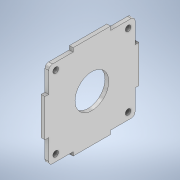
# Autodesk Inventor part: UpperSide
Saved by Autodesk Inventor 2022 (Build 260153000, 153)
## iProperties
Created: 2022-04-02
Part Number: UpperSide
Material: Aluminum 6061, Welded
Document SubType Name: Modeling
Designer: Sergei
Density: 2.7 g/cm^3
Appearance: Aluminum - Polished
Author: Sergei
Autodesk Inventor part; units mm, degrees
ref_plane "YZ Plane" through (0, 0, 0) normal (1, 0, 0) x (0, 1, 0)
ref_plane "XZ Plane" through (0, 0, 0) normal (0, 1, 0) x (-1, 0, 0)
ref_plane "XY Plane" through (0, 0, 0) normal (0, 0, 1) x (1, 0, 0)
sketch "Sketch1" plane through (0, 0, 0) normal (1, 0, 0) x (0, 1, 0)
  line L0 (-25, -25) -> (25, -25)
  line L1 (25, -25) -> (25, 25)
  line L2 (25, 25) -> (-25, 25)
  line L3 (-25, 25) -> (-25, -25)
  line L4 (-25, -25) -> (25, 25) construction
  line L5 (25, -25) -> (-25, 25) construction
  line L6 (-24, -24) -> (24, -24)
  line L7 (24, -24) -> (24, 24)
  line L8 (24, 24) -> (-24, 24)
  line L9 (-24, 24) -> (-24, -24)
  line L10 (-24, -24) -> (24, 24) construction
  line L11 (24, -24) -> (-24, 24) construction
  point P0 (0, 0)
  dimension "d0" = 50
  dimension "d1" = 50
  dimension "d2" = 48
  dimension "d3" = 48
  constraints: 24 end point, 4 midpoint, 4 parallel, 2 horizontal, 2 perpendicular, 1 point on line
  measures "d0" distance of L0.end L1.end
  measures "d1" distance of L0.start L0.end
  measures "d2" distance of L6.end L7.end
  measures "d3" distance of L6.start L6.end
extrude "Extrusion1" add sketch "Sketch1" along normal blind 2 contours L3 L2 L1 L0 | L9 L8 L7 L6
sketch "Sketch3" plane through (0, 0, 0) normal (-1, 0, 0) x (0, 0, 1)
  line L0 (19.3, -19.3) -> (-19.3, -19.3)
  line L1 (-19.3, -19.3) -> (-19.3, 19.3)
  line L2 (-19.3, 19.3) -> (19.3, 19.3)
  line L3 (19.3, 19.3) -> (19.3, -19.3)
  line L4 (19.3, -19.3) -> (-19.3, 19.3) construction
  line L5 (-19.3, -19.3) -> (19.3, 19.3) construction
  circle A0 centre (-19.3, 19.3) radius 1.5
  circle A1 centre (19.3, 19.3) radius 1.5555
  circle A2 centre (19.3, -19.3) radius 1.5555
  circle A3 centre (-19.3, -19.3) radius 1.5555
  point P0 (0, 0)
  dimension "d6" = 38.6
  dimension "d7" = 38.6
  dimension "d8" = 3
  dimension "d9" = 3.111
  dimension "d10" = 3.111
  dimension "d11" = 3.111
  constraints: 12 end point, 4 centre point, 4 coincident, 2 midpoint, 2 parallel, 1 horizontal, 1 perpendicular
  measures "d6" distance of L1.end L2.end
  measures "d7" distance of L2.end L0.start
  measures "d8" diameter of A0
  measures "d9" diameter of A1
  measures "d10" diameter of A2
  measures "d11" diameter of A3
hole "Hole1" at (0, 19.3, -19.3) direction (1, 0, 0) diameter 3 end through all
sketch "Sketch4" plane through (0, 0, 0) normal (-1, 0, 0) x (0, 0, 1)
  line L0 (-19.3, -19.3) -> (19.3, -19.3)
  line L1 (19.3, -19.3) -> (19.3, 19.3)
  line L2 (19.3, 19.3) -> (-19.3, 19.3)
  line L3 (-19.3, 19.3) -> (-19.3, -19.3)
  line L4 (-19.3, -19.3) -> (19.3, 19.3) construction
  line L5 (19.3, -19.3) -> (-19.3, 19.3) construction
  circle A0 centre (19.3, 19.3) radius 1.5
  point P0 (0, 0)
  dimension "d19" = 38.6
  dimension "d20" = 38.6
  dimension "d21" = 3
  constraints: 12 end point, 2 midpoint, 2 parallel, 1 centre point, 1 horizontal, 1 perpendicular, 1 point on line
  measures "d19" distance of L0.end L1.end
  measures "d20" distance of L0.start L0.end
  measures "d21" diameter of A0
hole "Hole2" at (0, 19.3, 19.3) direction (1, 0, 0) diameter 3 end through all
sketch "Sketch5" plane through (0, 0, 0) normal (-1, 0, 0) x (0, 0, 1)
  line L0 (19.3, -19.3) -> (-19.3, -19.3)
  line L1 (-19.3, -19.3) -> (-19.3, 19.3)
  line L2 (-19.3, 19.3) -> (19.3, 19.3)
  line L3 (19.3, 19.3) -> (19.3, -19.3)
  line L4 (19.3, -19.3) -> (-19.3, 19.3) construction
  line L5 (-19.3, -19.3) -> (19.3, 19.3) construction
  circle A0 centre (-19.3, -19.3) radius 1.5
  point P0 (0, 0)
  dimension "d29" = 38.6
  dimension "d30" = 38.6
  dimension "d31" = 3
  constraints: 12 end point, 2 midpoint, 2 parallel, 1 centre point, 1 coincident, 1 horizontal, 1 perpendicular
  measures "d29" distance of L1.end L2.end
  measures "d30" distance of L2.end L0.start
  measures "d31" diameter of A0
hole "Hole3" at (0, -19.3, -19.3) direction (1, 0, 0) diameter 3 end through all
sketch "Sketch6" plane through (0, 0, 0) normal (-1, 0, 0) x (0, 0, 1)
  line L0 (19.3, -19.3) -> (-19.3, -19.3)
  line L1 (-19.3, -19.3) -> (-19.3, 19.3)
  line L2 (-19.3, 19.3) -> (19.3, 19.3)
  line L3 (19.3, 19.3) -> (19.3, -19.3)
  line L4 (19.3, -19.3) -> (-19.3, 19.3) construction
  line L5 (-19.3, -19.3) -> (19.3, 19.3) construction
  circle A0 centre (19.3, -19.3) radius 1.5
  point P0 (0, 0)
  dimension "d39" = 38.6
  dimension "d40" = 38.6
  dimension "d41" = 3
  constraints: 12 end point, 2 midpoint, 2 parallel, 1 centre point, 1 coincident, 1 horizontal, 1 perpendicular
  measures "d39" distance of L1.end L2.end
  measures "d40" distance of L2.end L0.start
  measures "d41" diameter of A0
hole "Hole4" at (0, -19.3, 19.3) direction (1, 0, 0) diameter 3 end through all
sketch "Sketch7" plane through (0, 0, 0) normal (-1, 0, 0) x (0, 0, 1)
  line L0 (23, -23) -> (-23, -23)
  line L1 (-23, -23) -> (-23, 23)
  line L2 (-23, 23) -> (23, 23)
  line L3 (23, 23) -> (23, -23)
  line L4 (23, -23) -> (-23, 23) construction
  line L5 (-23, -23) -> (23, 23) construction
  line L6 (-25, 25) -> (25, 25) projected
  line L7 (10, 21) -> (-10, 21)
  line L8 (-10, 21) -> (-10, 25)
  line L9 (-10, 25) -> (10, 25)
  line L10 (10, 25) -> (10, 21)
  line L11 (10, 21) -> (-10, 25) construction
  line L12 (-10, 21) -> (10, 25) construction
  line L13 (21, -10) -> (25, -10)
  line L14 (25, -10) -> (25, 10)
  line L15 (25, 10) -> (21, 10)
  line L16 (21, 10) -> (21, -10)
  line L17 (21, -10) -> (25, 10) construction
  line L18 (25, -10) -> (21, 10) construction
  line L19 (25, -25) -> (-25, -25) projected
  line L20 (-10, -21) -> (10, -21)
  line L21 (10, -21) -> (10, -25)
  line L22 (10, -25) -> (-10, -25)
  line L23 (-10, -25) -> (-10, -21)
  line L24 (-10, -21) -> (10, -25) construction
  line L25 (10, -21) -> (-10, -25) construction
  line L26 (-25.0252, 10) -> (-20.9748, 10)
  line L27 (-20.9748, 10) -> (-20.9748, -10)
  line L28 (-20.9748, -10) -> (-25.0252, -10)
  line L29 (-25.0252, -10) -> (-25.0252, 10)
  line L30 (-25.0252, 10) -> (-20.9748, -10) construction
  line L31 (-20.9748, 10) -> (-25.0252, -10) construction
  line L32 (25, -25) -> (-25, -25)
  line L33 (-25, -25) -> (-25, 25)
  line L34 (-25, 25) -> (25, 25)
  line L35 (25, 25) -> (25, -25)
  line L36 (25, -25) -> (-25, 25) construction
  line L37 (-25, -25) -> (25, 25) construction
  point P0 (0, 0)
  point P1 (0, 23)
  point P2 (23, 0)
  point P3 (0, -23)
  point P4 (-23, 0)
  point P5 (-10, 23)
  point P6 (10, 23)
  point P7 (23, 10)
  point P8 (23, -10)
  point P9 (10, -23)
  point P10 (-10, -23)
  point P11 (-23, -10)
  point P12 (-23, 10)
  point P13 (10, 25)
  point P14 (-25, 10)
  point P15 (-25, -10)
  point P16 (-10, -25)
  dimension "d49" = 46
  dimension "d50" = 46
  dimension "d51" = 20
  dimension "d52" = 20
  dimension "d53" = 20
  dimension "d54" = 20
  constraints: 72 end point, 16 midpoint, 12 parallel, 6 horizontal, 6 perpendicular, 2 point on line
  measures "d49" distance of L1.end L2.end
  measures "d50" distance of L2.end L0.start
  measures "d51" distance of L7.start L7.end
  measures "d52" distance of L15.end L13.start
  measures "d53" distance of L20.start L20.end
  measures "d54" distance of L26.end L27.end
extrude "Extrusion3" cut sketch "Sketch7" against normal blind 2 contours L3 L13 L35 L19 L21 L0 | L23 L19 L33 L28 L1 L0 | L3 L2 L10 L6 L35 L15 | L26 L33 L6 L8 L2 L1
sketch "Sketch8" plane through (2, 0, 0) normal (1, 0, 0) x (0, 0, -1)
  circle A0 centre (0, 0) radius 9
  dimension "d59" = 18
  constraints: 1 centre point, 1 coincident
  measures "d59" diameter of A0
extrude "Extrusion4" cut sketch "Sketch8" against normal blind 2
sketch "Sketch9" plane through (2, 0, 0) normal (1, 0, 0) x (0, 0, -1)
  line L0 (13.75, -13.75) -> (-13.75, -13.75)
  line L1 (-13.75, -13.75) -> (-13.75, 13.75)
  line L2 (-13.75, 13.75) -> (13.75, 13.75)
  line L3 (13.75, 13.75) -> (13.75, -13.75)
  line L4 (13.75, -13.75) -> (-13.75, 13.75) construction
  line L5 (-13.75, -13.75) -> (13.75, 13.75) construction
  circle A0 centre (-13.75, 13.75) radius 1
  circle A1 centre (13.75, 13.75) radius 1
  circle A2 centre (13.75, -13.75) radius 1
  circle A3 centre (-13.75, -13.75) radius 1
  point P0 (0, 0)
  dimension "d62" = 27.5
  dimension "d63" = 27.5
  dimension "d64" = 2
  dimension "d65" = 2
  dimension "d66" = 2
  dimension "d67" = 2
  constraints: 12 end point, 4 centre point, 4 coincident, 2 midpoint, 2 parallel, 1 horizontal, 1 perpendicular
  measures "d62" distance of L1.end L2.end
  measures "d63" distance of L0.end L1.end
  measures "d64" diameter of A0
  measures "d65" diameter of A1
  measures "d66" diameter of A2
  measures "d67" diameter of A3
extrude "Extrusion5" [suppressed]
fillet "Fillet1" radius 2 4 edges at (1, 23, 23) (1, -23, 23) (1, -23, -23) (1, 23, -23)
body "Solid1"
